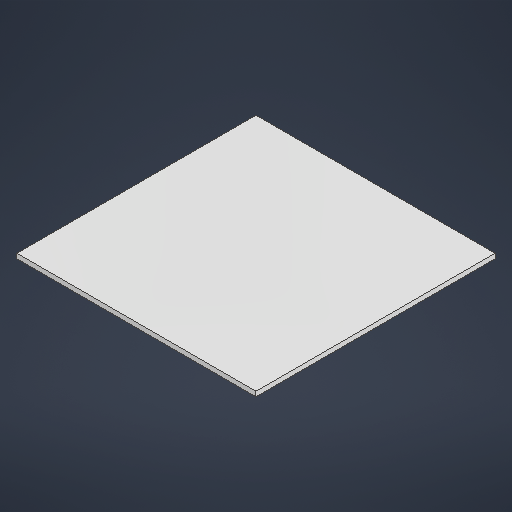
# Autodesk Inventor part: base
Saved by Autodesk Inventor 2026.2 (Build 302298010, 298A)
## iProperties
Created: 2026-03-01
Part Number: base
Material: Wood (Birch)
Document SubType Name: Modeling
Designer: Luke
Density: 0.55 g/cm^3
Appearance: Knurled 45
Author: Luke
Autodesk Inventor part; units mm, degrees
ref_plane "YZ Plane" through (0, 0, 0) normal (1, 0, 0) x (0, 1, 0)
ref_plane "XZ Plane" through (0, 0, 0) normal (0, 1, 0) x (-1, 0, 0)
ref_plane "XY Plane" through (0, 0, 0) normal (0, 0, 1) x (1, 0, 0)
sketch "Sketch1" plane through (0, 0, 0) normal (0, 1, 0) x (-1, 0, 0)
  line L0 (-250, -250) -> (250, -250)
  line L1 (250, -250) -> (250, 250)
  line L2 (250, 250) -> (-250, 250)
  line L3 (-250, 250) -> (-250, -250)
  line L4 (-250, -250) -> (250, 250) construction
  line L5 (250, -250) -> (-250, 250) construction
  point P0 (0, 0)
  dimension "d0" = 500
  dimension "d1" = 500
  constraints: 12 end point, 2 midpoint, 2 parallel, 1 horizontal, 1 perpendicular
  measures "d0" distance of L2.end L1.end
  measures "d1" distance of L1.end L0.end
extrude "Extrusion1" add sketch "Sketch1" along normal blind 10
sketch "Sketch2" plane through (0, 10, 0) normal (0, 1, 0) x (1, 0, 0)
  line L0 (225, -225) -> (-225, -225)
  line L1 (-225, -225) -> (-225, 225)
  line L2 (-225, 225) -> (225, 225)
  line L3 (225, 225) -> (225, -225)
  line L4 (225, -225) -> (-225, 225) construction
  line L5 (-225, -225) -> (225, 225) construction
  circle A0 centre (0, 0) radius 106.4612 construction
  dimension "d4" = 450
  dimension "d5" = 450
  constraints: 12 end point, 5 coincident, 2 midpoint, 2 parallel, 1 centre point, 1 horizontal, 1 perpendicular
  measures "d4" distance of L1.end L2.end
  measures "d5" distance of L0.end L1.end
body "Solid1"
